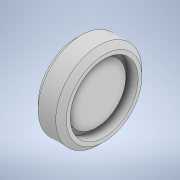
# Autodesk Inventor part: 711127
Saved by Autodesk Inventor 2022 (Build 260153000, 153)
## iProperties
Created: 2021-10-22
Part Number: 711127
Material: Типовые
Document SubType Name: Modeling
Designer: RaNSiD
Density: 1 g/cm^3
Appearance: По умолчанию
Author: RaNSiD
Autodesk Inventor part; units mm, degrees
ref_plane "YZ Plane" through (0, 0, 0) normal (1, 0, 0) x (0, 1, 0)
ref_plane "XZ Plane" through (0, 0, 0) normal (0, 1, 0) x (-1, 0, 0)
ref_plane "XY Plane" through (0, 0, 0) normal (0, 0, 1) x (1, 0, 0)
sketch "Эскиз1" plane through (0, 0, 0) normal (0, 0, 1) x (1, 0, 0)
  line L0 (0, 0) -> (0, 20)
  line L1 (0, 20) -> (2.8284, 22.8284)
  line L2 (0, 0) -> (15, 0)
  line L3 (15, 0) -> (15, 20)
  line L4 (15, 20) -> (12.1716, 22.8284)
  line L5 (12.1716, 22.8284) -> (2.8284, 22.8284)
  dimension "d0" = 20
  dimension "d1" = 4
  dimension "d2" = 135
  dimension "d3" = 15
  dimension "d4" = 4
  dimension "d5" = 135
  constraints: 12 end point, 1 horizontal, 1 parallel, 1 perpendicular, 1 vertical
  measures "d0" distance of L0.start L0.end
  measures "d1" distance of L0.end L1.end
  measures "d2" angle of L0 L1
  measures "d3" distance of L0.start L2.end
  measures "d4" distance of L3.end L4.end
  measures "d5" angle of L4 L3
revolve "Вращение1" add sketch "Эскиз1" angle 360 about axis through (0, 0, 0) along (1, 0, 0)
sketch "Эскиз2" plane through (0, 0, 0) normal (0, 0, 1) x (1, 0, 0)
  line L0 (15, -20) -> (15, 20) construction
  line L1 (15, 18) -> (9, 18)
  line L2 (9, 18) -> (9, 15.5)
  line L3 (9, 15.5) -> (11, 15.5)
  line L4 (11, 15.5) -> (11, 0)
  line L5 (11, 0) -> (15, 0)
  line L6 (15, 18) -> (15, 0)
  line L7 (0, -20) -> (0, 20) construction
  line L8 (0, 3) -> (4.5, 3)
  line L9 (4.5, 3) -> (4.5, 0)
  line L10 (4.5, 0) -> (0, 0)
  line L11 (0, 3) -> (0, 0)
  line L12 (0, 0) -> (15, 0)
  dimension "d7" = 4.5
  dimension "d8" = 3
  dimension "d9" = 18
  dimension "d10" = 15.5
  dimension "d11" = 4
  dimension "d12" = 6
  constraints: 22 end point, 7 perpendicular, 3 point on line, 2 horizontal, 1 collinear, 1 midpoint
  measures "d7" distance of L8.start L8.end
  measures "d8" distance of L8.end L9.end
  measures "d9" distance between parallel lines of L5 L1
  measures "d10" distance of L3.end L4.end
  measures "d11" distance of L4.end L5.end
  measures "d12" distance between parallel lines of L0 L2
revolve "Вращение2" cut sketch "Эскиз2" angle 360 about axis through (0, 0, 0) along (1, 0, 0)
